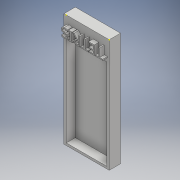
# Autodesk Inventor part: Tertrisgrej
Saved by Autodesk Inventor 2018 (Build 220112000, 112)
## iProperties
Created: 2017-12-01
Part Number: Tertrisgrej
Material: Generic
Document SubType Name: Modeling
Designer: 17riwi
Density: 1 g/cm^3
Appearance: Default
Author: 17riwi
Autodesk Inventor part; units mm, degrees
ref_plane "YZ Plane" through (0, 0, 0) normal (1, 0, 0) x (0, 1, 0)
ref_plane "XZ Plane" through (0, 0, 0) normal (0, 1, 0) x (-1, 0, 0)
ref_plane "XY Plane" through (0, 0, 0) normal (0, 0, 1) x (1, 0, 0)
sketch "Sketch1" plane through (0, 0, 0) normal (0, 1, 0) x (-1, 0, 0)
  line L0 (0, 0) -> (20, 0)
  line L1 (20, 0) -> (20, -50)
  line L2 (20, -50) -> (0, -50)
  line L3 (0, -50) -> (0, 0)
  line L4 (1, -49) -> (19, -49)
  line L5 (19, -49) -> (19, -9)
  line L6 (19, -9) -> (1, -9)
  line L7 (1, -9) -> (1, -49)
  line L8 (16.8025, -6.0734) -> (3.0569, -6.0734) construction
  line L9 (3.0569, -6.0734) -> (3.0569, -2.9167) construction
  line L10 (3.0569, -2.9167) -> (16.8025, -2.9167) construction
  line L11 (16.8025, -2.9167) -> (16.8025, -6.0734) construction
  constraints: 16 end point, 4 parallel, 2 horizontal, 2 perpendicular, 2 other
extrude "Extrusion1" add sketch "Sketch1" along normal blind 5
sketch "Sketch2" plane through (-19, 0, -49) normal (1, 0, 0) x (0, 0, -1)
  point P0 (-49, 0)
sketch "Sketch3" plane through (0, 5, 0) normal (0, 1, 0) x (1, 0, 0)
  line L0 (-1, 9) -> (-19, 9) projected
  line L1 (-1, 9) -> (-19, 9)
  line L2 (-19, 9) -> (-19, 49)
  line L3 (-19, 49) -> (-1, 49)
  line L4 (-1, 49) -> (-1, 9)
  point P0 (0, 0)
  constraints: 8 end point, 2 parallel, 1 horizontal, 1 perpendicular
extrude "Extrusion2" add sketch "Sketch3" against normal blind 1
sketch "Sketch4" plane through (0, 0, 0) normal (0, -1, 0) x (1, 0, 0)
  line L0 (-0.8346, -7.4271) -> (-19.3244, -7.4271) construction
  line L1 (-19.3244, -7.4271) -> (-19.3244, -3.1809) construction
  line L2 (-19.3244, -3.1809) -> (-0.8346, -3.1809) construction
  line L3 (-0.8346, -3.1809) -> (-0.8346, -7.4271) construction
  line L4 (-0.8346, -7.3351) -> (-4.0956, -7.3351)
  line L5 (-4.0956, -6.8858) -> (-2.7339, -6.8858)
  line L6 (-2.7339, -6.8858) -> (-2.7339, -3.2639)
  line L7 (-2.7339, -3.2639) -> (-2.1864, -3.2639)
  line L8 (-2.1864, -3.2639) -> (-2.1864, -6.8858)
  line L9 (-2.1864, -6.8858) -> (-0.8346, -6.8858)
  line L10 (-0.8346, -7.3351) -> (-4.0956, -7.3351)
  line L11 (-4.0956, -7.3351) -> (-4.0956, -6.8858)
  line L12 (-4.5589, -7.3351) -> (-7.0858, -7.3351)
  line L13 (-7.0858, -7.3351) -> (-7.0858, -6.8858)
  line L14 (-7.0858, -6.8858) -> (-5.0924, -6.8858)
  line L15 (-5.0924, -6.8858) -> (-5.0924, -5.7487)
  line L16 (-5.0924, -5.7487) -> (-6.9174, -5.7487)
  line L17 (-6.9174, -5.7487) -> (-6.9174, -5.304)
  line L18 (-6.9174, -5.304) -> (-5.0924, -5.304)
  line L19 (-5.0924, -5.304) -> (-5.0924, -3.7553)
  line L20 (-5.0924, -3.7553) -> (-7.0858, -3.7553)
  line L21 (-7.0858, -3.7553) -> (-7.0858, -3.2639)
  line L22 (-7.0858, -3.2639) -> (-4.5589, -3.2639)
  line L23 (-4.5589, -3.2639) -> (-4.5589, -7.3351)
  line L24 (-7.2683, -7.3351) -> (-7.2683, -6.8858)
  line L25 (-7.2683, -6.8858) -> (-8.6581, -6.8858)
  line L26 (-8.6581, -6.8858) -> (-8.6581, -3.2639)
  line L27 (-8.6581, -3.2639) -> (-9.2056, -3.2639)
  line L28 (-9.2056, -3.2639) -> (-9.2056, -6.8858)
  line L29 (-9.2056, -6.8858) -> (-10.5674, -6.8858)
  line L30 (-10.5674, -6.8858) -> (-10.5674, -7.3351)
  line L31 (-10.5674, -7.3351) -> (-7.2683, -7.3351)
  arc A0 (-12.2239, -5.2995) -> (-12.252, -6.8858) centre (-12.2118, -6.0931) ccw
  line L32 (-12.2239, -5.2995) -> (-11.536, -5.2995)
  line L33 (-11.536, -5.2995) -> (-11.536, -6.8858)
  line L34 (-11.536, -6.8858) -> (-12.1715, -6.8858)
  line L35 (-12.1715, -6.8858) -> (-12.252, -6.8858)
  line L36 (-11, -7.3351) -> (-11, -3.2639)
  line L37 (-11, -3.2639) -> (-11.536, -3.2639)
  line L38 (-11.536, -3.2639) -> (-11.536, -4.8924)
  line L39 (-11.536, -4.8924) -> (-12.1715, -4.8924)
  line L40 (-12.1715, -4.8924) -> (-13.4593, -3.2639)
  line L41 (-13.4593, -3.2639) -> (-14.1472, -3.2639)
  line L42 (-14.1472, -3.2639) -> (-12.7151, -5.0749)
  line L43 (-12.7151, -5.0749) -> (-14.1472, -3.2639)
  line L44 (-11, -7.3351) -> (-12.5187, -7.3351)
  arc A1 (-12.7151, -5.0749) -> (-12.5187, -7.3351) centre (-12.3177, -6.179) ccw
  line L45 (-2.2068, -3.254) -> (-2.2068, -6.869)
  line L46 (-2.2068, -6.869) -> (-0.8312, -6.869)
  line L47 (-0.8312, -6.869) -> (-0.8312, -7.354)
  line L48 (-0.8312, -7.354) -> (-4.1272, -7.354)
  line L49 (-4.1272, -7.354) -> (-4.1272, -6.869)
  line L50 (-4.1272, -6.869) -> (-2.7517, -6.869)
  line L51 (-2.7517, -6.869) -> (-2.7517, -3.254)
  line L52 (-2.7517, -3.254) -> (-2.2068, -3.254)
  line L53 (-4.5425, -3.254) -> (-4.5425, -7.354)
  line L54 (-4.5425, -7.354) -> (-7.1075, -7.354)
  line L55 (-7.1075, -7.354) -> (-7.1075, -6.869)
  line L56 (-7.1075, -6.869) -> (-5.0874, -6.869)
  line L57 (-5.0874, -6.869) -> (-5.0874, -5.7459)
  line L58 (-5.0874, -5.7459) -> (-6.9713, -5.7459)
  line L59 (-6.9713, -5.7459) -> (-6.9713, -5.2608)
  line L60 (-6.9713, -5.2608) -> (-5.0874, -5.2608)
  line L61 (-5.0874, -5.2608) -> (-5.0874, -3.7391)
  line L62 (-5.0874, -3.7391) -> (-7.1075, -3.7391)
  line L63 (-7.1075, -3.7391) -> (-7.1075, -3.254)
  line L64 (-7.1075, -3.254) -> (-4.5425, -3.254)
  line L65 (-8.6624, -3.254) -> (-8.6624, -6.869)
  line L66 (-8.6624, -6.869) -> (-7.2869, -6.869)
  line L67 (-7.2869, -6.869) -> (-7.2869, -7.354)
  line L68 (-7.2869, -7.354) -> (-10.5829, -7.354)
  line L69 (-10.5829, -7.354) -> (-10.5829, -6.869)
  line L70 (-10.5829, -6.869) -> (-9.2073, -6.869)
  line L71 (-9.2073, -6.869) -> (-9.2073, -3.254)
  line L72 (-9.2073, -3.254) -> (-8.6624, -3.254)
  line L73 (-14.1712, -3.254) -> (-13.4635, -3.254)
  line L74 (-13.4635, -3.254) -> (-12.1677, -4.8854)
  line L75 (-12.1677, -4.8854) -> (-11.5431, -4.8854)
  line L76 (-11.5431, -4.8854) -> (-11.5431, -3.254)
  line L77 (-11.5431, -3.254) -> (-10.9982, -3.254)
  line L78 (-10.9982, -3.254) -> (-10.9982, -7.354)
  line L79 (-10.9982, -7.354) -> (-12.0547, -7.354)
  spline S0 degree 2 poles (-12.0547, -7.354) (-12.4069, -7.354) (-12.8821, -7.2776) (-13.098, -7.1381) knots 0 0 0 1 2 2 2
  spline S1 degree 2 poles (-13.098, -7.1381) (-13.314, -6.9985) (-13.5632, -6.5633) (-13.5632, -6.241) knots 0 0 0 1 2 2 2
  spline S2 degree 2 poles (-13.5632, -6.241) (-13.5632, -5.7925) (-13.1047, -5.1844) (-12.7126, -5.0382) knots 0 0 0 1 2 2 2
  line L80 (-12.7126, -5.0382) -> (-14.1712, -3.254)
  spline S3 degree 2 poles (-12.995, -6.1978) (-12.995, -6.3772) (-12.8688, -6.653) (-12.7359, -6.7427) knots 0 0 0 1 2 2 2
  spline S4 degree 2 poles (-12.7359, -6.7427) (-12.6196, -6.8191) (-12.3106, -6.8822) (-12.0846, -6.8822) knots 0 0 0 1 2 2 2
  line L81 (-12.0846, -6.8822) -> (-11.5431, -6.8822)
  line L82 (-11.5431, -6.8822) -> (-11.5431, -5.3406)
  line L83 (-11.5431, -5.3406) -> (-12.0215, -5.3406)
  spline S5 degree 2 poles (-12.0215, -5.3406) (-12.2574, -5.3406) (-12.6329, -5.4237) (-12.7624, -5.5532) knots 0 0 0 1 2 2 2
  spline S6 degree 2 poles (-12.7624, -5.5532) (-12.8821, -5.6662) (-12.995, -5.9852) (-12.995, -6.1978) knots 0 0 0 1 2 2 2
  line L84 (-15.9255, -3.254) -> (-14.3373, -3.254)
  line L85 (-14.3373, -3.254) -> (-14.3373, -3.6727)
  line L86 (-14.3373, -3.6727) -> (-14.859, -3.6727)
  line L87 (-14.859, -3.6727) -> (-14.859, -6.9354)
  line L88 (-14.859, -6.9354) -> (-14.3373, -6.9354)
  line L89 (-14.3373, -6.9354) -> (-14.3373, -7.354)
  line L90 (-14.3373, -7.354) -> (-15.9255, -7.354)
  line L91 (-15.9255, -7.354) -> (-15.9255, -6.9354)
  line L92 (-15.9255, -6.9354) -> (-15.4039, -6.9354)
  line L93 (-15.4039, -6.9354) -> (-15.4039, -3.6727)
  line L94 (-15.4039, -3.6727) -> (-15.9255, -3.6727)
  line L95 (-15.9255, -3.6727) -> (-15.9255, -3.254)
  spline S7 degree 2 poles (-17.7429, -3.1809) (-17.2977, -3.1809) (-16.6731, -3.367) (-16.3973, -3.4999) knots 0 0 0 1 2 2 2
  line L96 (-16.3973, -3.4999) -> (-16.3973, -4.1843)
  line L97 (-16.3973, -4.1843) -> (-16.4372, -4.1843)
  spline S8 degree 2 poles (-16.4372, -4.1843) (-16.7063, -3.9318) (-17.3874, -3.6527) (-17.703, -3.6527) knots 0 0 0 1 2 2 2
  spline S9 degree 2 poles (-17.703, -3.6527) (-18.1549, -3.6527) (-18.6167, -4.0282) (-18.6167, -4.3372) knots 0 0 0 1 2 2 2
  spline S10 degree 2 poles (-18.6167, -4.3372) (-18.6167, -4.5831) (-18.3742, -4.8887) (-18.1117, -4.9651) knots 0 0 0 1 2 2 2
  spline S11 degree 2 poles (-18.1117, -4.9651) (-17.9223, -5.0183) (-17.6067, -5.0914) (-17.3708, -5.1512) knots 0 0 0 1 2 2 2
  spline S12 degree 2 poles (-17.3708, -5.1512) (-17.1581, -5.2077) (-16.8226, -5.3771) (-16.693, -5.5134) knots 0 0 0 1 2 2 2
  spline S13 degree 2 poles (-16.693, -5.5134) (-16.5667, -5.6496) (-16.4272, -6.0151) (-16.4272, -6.2543) knots 0 0 0 1 2 2 2
  spline S14 degree 2 poles (-16.4272, -6.2543) (-16.4272, -6.7527) (-17.2047, -7.4271) (-17.806, -7.4271) knots 0 0 0 1 2 2 2
  spline S15 degree 2 poles (-17.806, -7.4271) (-18.1516, -7.4271) (-18.7629, -7.2909) (-19.0254, -7.1613) knots 0 0 0 1 2 2 2
  line L98 (-19.0254, -7.1613) -> (-19.0254, -6.5101)
  line L99 (-19.0254, -6.5101) -> (-18.9855, -6.5101)
  spline S16 degree 2 poles (-18.9855, -6.5101) (-18.7895, -6.6895) (-18.1782, -6.9553) (-17.8426, -6.9553) knots 0 0 0 1 2 2 2
  spline S17 degree 2 poles (-17.8426, -6.9553) (-17.4638, -6.9553) (-16.9953, -6.5998) (-16.9953, -6.3108) knots 0 0 0 1 2 2 2
  spline S18 degree 2 poles (-16.9953, -6.3108) (-16.9953, -6.0516) (-17.2711, -5.7426) (-17.5303, -5.6728) knots 0 0 0 1 2 2 2
  spline S19 degree 2 poles (-17.5303, -5.6728) (-17.703, -5.6263) (-18.2047, -5.5067) (-18.3709, -5.4569) knots 0 0 0 1 2 2 2
  spline S20 degree 2 poles (-18.3709, -5.4569) (-18.7928, -5.3273) (-19.1849, -4.8057) (-19.1849, -4.4236) knots 0 0 0 1 2 2 2
  spline S21 degree 2 poles (-19.1849, -4.4236) (-19.1849, -4.181) (-18.9889, -3.7159) (-18.8128, -3.5531) knots 0 0 0 1 2 2 2
  spline S22 degree 2 poles (-18.8128, -3.5531) (-18.6167, -3.3737) (-18.1184, -3.1809) (-17.7429, -3.1809) knots 0 0 0 1 2 2 2
  point P0 (0, 0)
  constraints: 82 end point, 19 perpendicular, 18 point on line, 5 parallel, 4 point on circle, 3 collinear, 3 horizontal, 2 centre point, 2 vertical, 2 other
sketch "Sketch5" plane through (0, 0, 0) normal (0, -1, 0) x (1, 0, 0)
  point P0 (0, 0)
sketch "Sketch6" plane through (0, 0, 0) normal (0, -1, 0) x (1, 0, 0)
  line L0 (-19, -7) -> (-19, -6.5078)
  line L1 (-19, -6.5078) -> (-19, -7.1819)
  point P0 (0, 0)
  constraints: 4 end point, 1 point on line, 1 vertical
sketch "Sketch7" plane through (0, 0, 0) normal (0, -1, 0) x (1, 0, 0)
  point P0 (0, 0)
extrude "Extrusion3" add sketch "Sketch4" along normal blind 2 contours L45 L46 L47 L48 L49 L50 L51 L52 | L23 L22 L21 L62 L63 L64 L53 L54 L55 L56 L15 L14 L13 L12 | L12 L13 L14 L15 L56 L57 L58 L17 L18 L19 L60 L61 L62 L21 L22 L23 | L19 L18 L17 L58 L59 L60 | L67 L68 L69 L70 L28 L29 L30 L31 | L31 L30 L29 L28 L27 L65 L66 L26 L25 L67 | L25 L26 L66 L67 | L27 L71 L72 L65 | L32 L33 L34 L35 A0 S4 L81 L82 L83 S5 S6 S3 | L44 S0 A1 L42 S2 L80 L41 L40 L39 L38 L37 L36 | L78 L79 S0 L44 | L37 L38 L39 L40 L41 L42 L80 L73 L74 L75 L76 L77 L78 | S0 S1 S2 L42 A1 | L84 L85 L86 L87 L88 L89 L90 L91 L92 L93 L94 L95 | S7 L96 L97 S8 S9 S10 S11 S12 S13 S14 S15 L98 L99 S16 S17 S18 S19 S20 S21 S22
sketch "Sketch8" plane through (0, 0, 0) normal (0, -1, 0) x (1, 0, 0)
  point P0 (0, 0)
body "Solid1"
